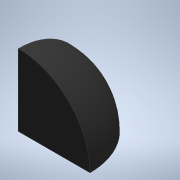
# Autodesk Inventor part: r_elbow
Saved by Autodesk Inventor 2021.1 (Build 251245010, 245A)
## iProperties
Created: 2017-07-18
Part Number: r_elbow
Material: ゴム
Document SubType Name: Modeling
Designer: gisen
Density: 0.93 g/cm^3
Appearance: ゴム - 黒
Author: gisen
Autodesk Inventor part; units mm, degrees
ref_plane "YZ Plane" through (0, 0, 0) normal (1, 0, 0) x (0, 1, 0)
ref_plane "XZ Plane" through (0, 0, 0) normal (0, 1, 0) x (-1, 0, 0)
ref_plane "XY Plane" through (0, 0, 0) normal (0, 0, 1) x (1, 0, 0)
sketch "スケッチ1" plane through (0, 0, 0) normal (0, 0, 1) x (1, 0, 0)
  arc A0 (20, 0) -> (0, 20) centre (0, 0) ccw
  line L0 (0, 0) -> (0, 20)
  line L1 (20, 0) -> (0, 0)
  dimension "d0" = 20
  constraints: 4 end point, 2 point on circle, 1 centre point, 1 coincident, 1 perpendicular, 1 vertical
  measures "d0" radius of A0
revolve "回転1" add sketch "スケッチ1" angle 90 about axis through (0, 0, 0) along (0, -1, 0)
